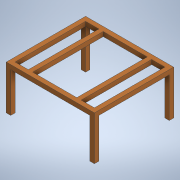
# Autodesk Inventor part: Game Desogn Truss
Saved by Autodesk Inventor 2021 (Build 250183000, 183)
## iProperties
Created: 2021-02-06
Part Number: Game Desogn Truss
Material: Iron, Gray
Document SubType Name: Modeling
Designer: aidan
Density: 7.15 g/cm^3
Appearance: Rust
Author: aidan
Autodesk Inventor part; units mm, degrees
ref_plane "YZ Plane" through (0, 0, 0) normal (1, 0, 0) x (0, 1, 0)
ref_plane "XZ Plane" through (0, 0, 0) normal (0, 1, 0) x (-1, 0, 0)
ref_plane "XY Plane" through (0, 0, 0) normal (0, 0, 1) x (1, 0, 0)
sketch "Sketch1" plane through (0, 0, 0) normal (0, 1, 0) x (-1, 0, 0)
  line L0 (-3048, 2743.2) -> (3048, 2743.2)
  line L1 (3048, 2743.2) -> (3048, -2743.2)
  line L2 (3048, -2743.2) -> (-3048, -2743.2)
  line L3 (-3048, -2743.2) -> (-3048, 2743.2)
  line L4 (-3048, 2743.2) -> (3048, -2743.2) construction
  line L5 (3048, 2743.2) -> (-3048, -2743.2) construction
  line L6 (2743.2, -2438.4) -> (2743.2, 2438.4)
  line L7 (-2743.2, 2438.4) -> (-2743.2, -2438.4)
  line L8 (1524, 2438.4) -> (1524, -2438.4)
  line L9 (1828.8, -2438.4) -> (1828.8, 2438.4)
  line L10 (-1524, -2438.4) -> (-1524, 2438.4)
  line L11 (-1828.8, 2438.4) -> (-1828.8, -2438.4)
  line L12 (1828.8, -2438.4) -> (2743.2, -2438.4)
  line L13 (-1828.8, 2438.4) -> (-2743.2, 2438.4)
  line L14 (-2743.2, -2438.4) -> (-1828.8, -2438.4)
  line L15 (-1524, -2438.4) -> (1524, -2438.4)
  line L16 (2743.2, 2438.4) -> (1828.8, 2438.4)
  line L17 (1524, 2438.4) -> (-1524, 2438.4)
  point P0 (0, 0)
  dimension "d0" = 6096
  dimension "d1" = 5486.4
  dimension "d3" = 304.8
  dimension "d4" = 914.4
  dimension "d5" = 914.4
  dimension "d6" = 304.8
  dimension "d7" = 304.8
  dimension "d8" = 304.8
  dimension "d10" = 304.8
  dimension "d11" = 304.8
  constraints: 36 end point, 14 parallel, 4 collinear, 4 perpendicular, 2 midpoint, 1 horizontal
  measures "d0" distance of L1.end L2.end
  measures "d1" distance between parallel lines of L0 L2
  measures "d3" distance between parallel lines of L11 L10
  measures "d4" distance between parallel lines of L7 L11
  measures "d5" distance between parallel lines of L6 L9
  measures "d6" distance between parallel lines of L2 L15
  measures "d7" distance between parallel lines of L8 L9
  measures "d8" distance between parallel lines of L3 L7
  measures "d10" distance between parallel lines of L0 L17
  measures "d11" distance between parallel lines of L1 L6
extrude "Extrusion1" add sketch "Sketch1" against normal blind 304.8
sketch "Sketch2" plane through (0, -304.8, 0) normal (0, -1, 0) x (1, 0, 0)
  line L0 (1828.8, -2438.4) -> (2743.2, -2438.4) projected
  line L1 (2743.2, -2438.4) -> (3048, -2438.4)
  line L2 (3048, -2438.4) -> (3048, -2743.2)
  line L3 (3048, -2743.2) -> (2743.2, -2743.2)
  line L4 (2743.2, -2743.2) -> (2743.2, -2438.4)
  line L5 (-1828.8, -2438.4) -> (-2743.2, -2438.4) projected
  line L6 (-3048, -2743.2) -> (3048, -2743.2) projected
  line L7 (-2743.2, -2438.4) -> (-3048, -2438.4)
  line L8 (-3048, -2438.4) -> (-3048, -2743.2)
  line L9 (-3048, -2743.2) -> (-2743.2, -2743.2)
  line L10 (-2743.2, -2743.2) -> (-2743.2, -2438.4)
  line L11 (-2743.2, -2438.4) -> (-2743.2, 2438.4) projected
  line L12 (3048, 2743.2) -> (-3048, 2743.2) projected
  line L13 (-2743.2, 2438.4) -> (-3048, 2438.4)
  line L14 (-3048, 2438.4) -> (-3048, 2743.2)
  line L15 (-3048, 2743.2) -> (-2743.2, 2743.2)
  line L16 (-2743.2, 2743.2) -> (-2743.2, 2438.4)
  line L17 (2743.2, 2438.4) -> (1828.8, 2438.4) projected
  line L18 (3048, 2743.2) -> (2743.2, 2743.2)
  line L19 (2743.2, 2743.2) -> (2743.2, 2438.4)
  line L20 (2743.2, 2438.4) -> (3048, 2438.4)
  line L21 (3048, 2438.4) -> (3048, 2743.2)
  point P0 (0, 0)
  constraints: 32 end point, 8 parallel, 4 horizontal, 4 perpendicular
extrude "Extrusion2" add sketch "Sketch2" along normal blind 2743.2
body "Solid1"
